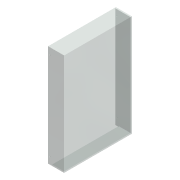
# Autodesk Inventor part: Стеклянная крышка
Saved by Autodesk Inventor 2022 (Build 260153000, 153)
## iProperties
Created: 2023-02-19
Part Number: Стеклянная крышка
Material: Типовые
Document SubType Name: Modeling
Designer: Глеб
Density: 1 g/cm^3
Appearance: Бесцветный
Author: Глеб
Autodesk Inventor part; units mm, degrees
ref_plane "YZ Plane" through (0, 0, 0) normal (1, 0, 0) x (0, 1, 0)
ref_plane "XZ Plane" through (0, 0, 0) normal (0, 1, 0) x (-1, 0, 0)
ref_plane "XY Plane" through (0, 0, 0) normal (0, 0, 1) x (1, 0, 0)
sketch "Эскиз1" plane through (0, 0, 0) normal (1, 0, 0) x (0, 1, 0)
  line L0 (-300, 200) -> (300, 200)
  line L1 (300, 200) -> (300, -200)
  line L2 (300, -200) -> (-300, -200)
  line L3 (-300, -200) -> (-300, 200)
  line L4 (-300, 200) -> (300, -200) construction
  line L5 (300, 200) -> (-300, -200) construction
  point P0 (0, 0)
  dimension "d0" = 400
  dimension "d1" = 600
  constraints: 12 end point, 2 midpoint, 2 parallel, 1 horizontal, 1 perpendicular
  measures "d0" distance of L0.end L1.end
  measures "d1" distance of L1.end L2.end
extrude "Выдавливание1" add sketch "Эскиз1" along normal blind 4
sketch "Эскиз2" plane through (0, 0, 0) normal (-1, 0, 0) x (0, 0, 1)
  line L0 (-200, -300) -> (-200, 300) projected
  line L1 (-200, 300) -> (200, 300) projected
  line L2 (-200, -300) -> (-196, -300)
  line L3 (-196, -300) -> (-196, 300)
  line L4 (-196, 300) -> (-200, 300)
  line L5 (-200, 300) -> (-200, -300)
  line L6 (200, 300) -> (200, -300) projected
  line L7 (-200, 300) -> (200, 300)
  line L8 (200, 300) -> (200, 296)
  line L9 (200, 296) -> (-200, 296)
  line L10 (-200, 296) -> (-200, 300)
  line L11 (200, -300) -> (196, -300)
  line L12 (196, -300) -> (196, 300)
  line L13 (196, 300) -> (200, 300)
  line L14 (200, 300) -> (200, -300)
  point P0 (0, 0)
  point P1 (-196, 296)
  point P2 (196, 296)
  dimension "d4" = 4
  dimension "d5" = 4
  dimension "d6" = 4
  constraints: 24 end point, 6 parallel, 5 point on line, 3 horizontal, 3 perpendicular
  measures "d4" distance between parallel lines of L0 L3
  measures "d5" distance between parallel lines of L1 L9
  measures "d6" distance between parallel lines of L6 L12
extrude "Выдавливание2" add sketch "Эскиз2" along normal blind 95
sketch "Эскиз3" plane through (0, 0, 0) normal (-1, 0, 0) x (0, 0, 1)
  line L0 (-200, 300) -> (-200, -300) projected
  line L1 (200, -300) -> (200, 300) projected
  line L2 (-200, -300) -> (200, -300)
  line L3 (200, -300) -> (200, -296)
  line L4 (200, -296) -> (-200, -296)
  line L5 (-200, -296) -> (-200, -300)
  point P0 (0, 0)
  point P1 (-200, -296)
  dimension "d10" = 4
  constraints: 8 end point, 2 parallel, 1 horizontal, 1 perpendicular, 1 point on line
  measures "d10" distance between parallel lines of L2 L4
extrude "Выдавливание3" add sketch "Эскиз3" along normal blind 70
sketch "Эскиз4" plane through (4, -300, -200) normal (0, 0, -1) x (-1, 0, 0)
  line L0 (4, 300) -> (99, 300) construction
  line L1 (99, 0) -> (99, 600) projected
  line L2 (0, 0) -> (99, 0) projected
  point P0 (89, 560)
  point P1 (89, 40)
  dimension "d13" = 10
  dimension "d14" = 40
  constraints: 2 end point, 1 midpoint, 1 symmetric about line
  measures "d13" distance from line of L1 point (89, 560)
  measures "d14" distance from line of L2 point (89, 40)
hole "Отверстие1" at (-85, 260, -200) at (-85, -260, -200) direction (0, 0, 1) diameter 3.9 depth 6 countersink diameter 4.5 countersink angle 90
sketch "Эскиз5" plane through (4, -300, 200) normal (0, 0, 1) x (1, 0, 0)
  circle A0 centre (-89, 560) radius 2.25 projected
  circle A1 centre (-89, 40) radius 2.25 projected
  point P0 (-4, 300)
hole "Отверстие2" at (-85, 260, 200) at (-85, -260, 200) direction (0, 0, -1) diameter 3.9 depth 6 countersink diameter 4 countersink angle 90
equation "\"d5\" = d4"
equation "\"d6\" = d4"
